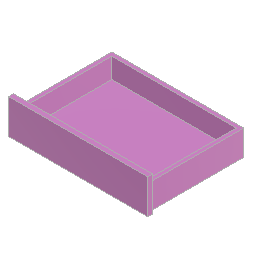
Drawer-Size-Reference (Autodesk Fusion 360 design; units mm, degrees)
Autodesk Fusion 360 part; units mm, degrees
sketch "Sketch1" plane through (0, 0, 0) normal (0, 0, 1) x (1, 0, 0)
  line L0 (0, 0) -> (407.924, 0)
  line L1 (407.924, 0) -> (407.924, -297.942)
  line L2 (407.924, -297.942) -> (0, -297.942)
  line L3 (0, -297.942) -> (0, 0)
  dimension "d1" = 407.924
  dimension "d2" = 297.942
  constraint horizontal L0
  constraint vertical L1
  constraint horizontal L2
  constraint vertical L3
  constraint coincident L0.start L3.end
  measures "d1" distance of L0.start L0.end
  measures "d2" distance of L0.start L2.end
extrude "Extrude1" add sketch "Sketch1" along normal blind 3.175
sketch "Sketch2" plane through (0, 0, 3.175) normal (0, 0, 1) x (-1, 0, 0)
  line L0 (0, 297.942) -> (-407.924, 297.942)
  line L1 (-407.924, 297.942) -> (-407.924, 0)
  line L2 (-407.924, 0) -> (0, 0)
  line L3 (0, 0) -> (0, 297.942)
  line L4 (-420.074, 297.942) -> (-420.074, -12.15)
  line L5 (-420.074, -12.15) -> (12.15, -12.15)
  line L6 (12.15, -12.15) -> (12.15, 297.942)
  line L7 (0, 297.942) -> (12.15, 297.942)
  line L8 (12.15, 297.942) -> (-420.074, 297.942)
  constraint coincident L0.start L3.end
  constraint perpendicular L6 L7
  constraint perpendicular L4 L8
extrude "Extrude2" add sketch "Sketch2" against normal blind 17 contours L1 L2 L3 L4 L5 L6 L7 L8
sketch "Sketch3" plane through (0, 0, 3.175) normal (0, 0, 1) x (-1, 0, 0)
  line L0 (12.15, 297.942) -> (-420.074, 297.942)
  line L1 (-420.074, 297.942) -> (-420.074, -12.15)
  line L2 (-420.074, -12.15) -> (12.15, -12.15)
  line L3 (12.15, -12.15) -> (12.15, 297.942)
  line L4 (-407.924, 285.792) -> (-407.924, 0)
  line L5 (-407.924, 0) -> (0, 0)
  line L6 (0, 0) -> (0, 285.792)
  line L7 (0, 285.792) -> (-407.924, 285.792)
  line L8 (0, 285.792) -> (0, 297.942)
  line L9 (-407.924, 285.792) -> (-407.924, 297.942)
  line L10 (-407.924, 297.942) -> (0, 297.942)
  line L11 (0, 297.942) -> (12.15, 297.942)
  line L12 (12.15, 297.942) -> (12.15, -12.15)
  line L13 (12.15, -12.15) -> (0, -12.15)
  line L14 (-420.074, -12.15) -> (-420.074, 297.942)
  line L15 (-420.074, 297.942) -> (-407.924, 297.942)
  line L16 (-420.074, -12.15) -> (12.15, -12.15)
  dimension "d8" = -12.15
  constraint coincident L0 L8.end
  constraint perpendicular L0 L8
  constraint coincident L0 L9.end
  constraint perpendicular L0 L9
  constraint coincident L0.start L3.end
  constraint coincident L2.end L3.start
  constraint coincident L2 L13.end
  constraint coincident L1.end L2.start
  constraint coincident L0.end L1.start
extrude "Extrude3" add sketch "Sketch3" along normal blind 66.15 contours L0 L1 L2 L3 L4 L5 L6 L8 L9 L11 L12 L13 L14 L15 L16
sketch "Sketch4" plane through (0, 0, -13.825) normal (0, 0, -1) x (1, 0, 0)
  line L0 (420.074, 297.942) -> (407.924, 297.942)
  line L1 (407.924, 297.942) -> (407.924, 0)
  line L2 (407.924, 0) -> (0, 0)
  line L3 (0, 0) -> (0, 297.942)
  line L4 (0, 297.942) -> (-12.15, 297.942)
  line L5 (-12.15, 297.942) -> (-12.15, -12.15)
  line L6 (-12.15, -12.15) -> (420.074, -12.15)
  line L7 (420.074, -12.15) -> (420.074, 297.942)
  line L8 (-12.15, 297.942) -> (-23.9, 297.942)
  line L9 (420.074, 297.942) -> (431.824, 297.942)
  line L10 (-23.9, 297.942) -> (-23.9, 313.942)
  line L11 (431.824, 297.942) -> (431.824, 313.942)
  line L12 (-23.9, 313.942) -> (431.824, 313.942)
  line L13 (-12.15, 297.942) -> (420.074, 297.942)
  dimension "d11" = 11.75
  dimension "d12" = 11.75
  dimension "d14" = 16
  dimension "d15" = 16
  constraint coincident L4.end L5.start
  constraint perpendicular L5 L8
  constraint coincident L0.start L7.end
  constraint perpendicular L7 L9
  constraint perpendicular L8 L10
  constraint perpendicular L9 L11
  measures "d11" distance of L4.end L8.end
  measures "d12" distance of L0.start L9.end
  measures "d14" distance of L8.end L10.end
  measures "d15" distance of L9.end L11.end
extrude "Extrude4" add sketch "Sketch4" against normal blind 113.5 contours L0 L4 L8 L9 L10 L11 L12 L13
